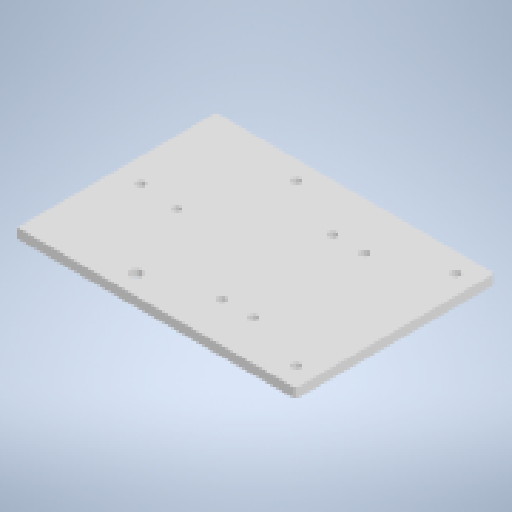
# Autodesk Inventor part: C beam gantry (big side y axis)
Saved by Autodesk Inventor 2023.2 (Build 272271000, 271)
## iProperties
Created: 2023-03-20
Part Number: C beam gantry (big side y axis)
Material: Generic
Document SubType Name: Modeling
Designer: dmargari
Density: 1 g/cm^3
Appearance: Default
Author: dmargari
Autodesk Inventor part; units mm, degrees
ref_plane "YZ Plane" through (0, 0, 0) normal (1, 0, 0) x (0, 1, 0)
ref_plane "XZ Plane" through (0, 0, 0) normal (0, 1, 0) x (-1, 0, 0)
ref_plane "XY Plane" through (0, 0, 0) normal (0, 0, 1) x (1, 0, 0)
sketch "Sketch1" plane through (0, 0, 0) normal (0, 1, 0) x (-1, 0, 0)
  line L0 (185.292, -262.2018) -> (60.092, -262.2018)
  line L1 (60.092, -262.2018) -> (60.092, -387.4018)
  line L2 (60.092, -387.4018) -> (185.292, -387.4018)
  line L3 (185.292, -387.4018) -> (185.292, -262.2018) construction
  line L4 (172.992, -262.2018) -> (172.992, -387.4018) construction
  line L5 (72.392, -262.2018) -> (72.392, -387.4018) construction
  line L6 (185.292, -262.2018) -> (235.292, -262.2018)
  line L7 (235.292, -262.2018) -> (235.292, -387.4018)
  line L8 (235.292, -387.4018) -> (185.292, -387.4018)
  line L9 (197.26, -375.1018) -> (25.4497, -375.1018) construction
  line L10 (197.26, -274.5018) -> (25.4497, -274.5018) construction
  point P0 (0, 0)
  point P1 (-73.8984, 140.5937)
  point P2 (172.992, -375.1018)
  point P3 (72.392, -375.1018)
  point P4 (172.992, -274.5018)
  point P5 (72.392, -274.5018)
  dimension "d0" = 125.2
  dimension "d1" = 125.2
  dimension "d2" = 12.3
  dimension "d3" = 12.3
  dimension "d8" = 50
  dimension "d35" = 12.3
  dimension "d36" = 100.6
  constraints: 22 end point, 13 point on line, 4 horizontal, 4 perpendicular, 2 parallel, 1 collinear
  measures "d0" distance of L2.end L1.end
  measures "d1" distance of L1.end L0.end
  measures "d2" distance between parallel lines of L1 L5
  measures "d3" distance between parallel lines of L3 L4
  measures "d8" distance of L0.start L6.end
  measures "d35" distance between parallel lines of L2 L9
  measures "d36" distance between parallel lines of L9 L10
extrude "Extrusion1" add sketch "Sketch1" along normal blind 6
fillet "Fillet1" radius 2 2 edges at (-60.092, 3, -262.2018) (-60.092, 3, -387.4018)
sketch "Sketch2" plane through (0, 6, 0) normal (0, 1, 0) x (1, 0, 0)
  line L0 (-235.292, 387.4018) -> (-235.292, 262.2018) construction
  line L1 (-235.292, 324.8018) -> (-60.092, 324.8018) construction
  line L2 (-60.092, 264.2018) -> (-60.092, 385.4018) construction
  line L3 (-235.192, 314.8018) -> (-30.192, 314.8018) construction
  line L4 (-235.192, 334.8018) -> (-30.192, 334.8018) construction
  line L5 (-235.292, 262.2018) -> (-62.092, 262.2018) construction
  line L6 (-220.292, 262.2018) -> (-220.292, 387.4018) construction
  line L7 (-62.092, 387.4018) -> (-235.292, 387.4018) construction
  line L8 (-195.292, 257.4018) -> (-195.292, 387.4018) construction
  point P0 (0, 0)
  point P1 (-220.292, 324.8018)
  point P2 (-195.292, 322.4018)
  dimension "d12" = 10
  dimension "d13" = 10
  dimension "d14" = 15
  dimension "d15" = 25
  constraints: 10 end point, 4 midpoint, 2 parallel, 2 point on line, 2 vertical
  measures "d12" distance between parallel lines of L1 L3
  measures "d13" distance between parallel lines of L1 L4
  measures "d14" distance between parallel lines of L0 L6
  measures "d15" distance between parallel lines of L8 L6
hole "Hole1" at (-220.292, 6, -324.8018) at (-195.292, 6, -322.4018) direction (0, -1, 0) diameter 5.1 end through all
sketch "Sketch3" plane through (0, 6, 0) normal (0, 1, 0) x (1, 0, 0)
  circle A0 centre (-112.092, 292.2018) radius 2.55 projected
  circle A1 centre (-132.092, 292.2018) radius 2.55 projected
  circle A2 centre (-132.092, 357.4018) radius 2.55 projected
  circle A3 centre (-112.092, 357.4018) radius 2.55 projected
  point P0 (0, 0)
hole "Hole2" at (-132.092, 6, -292.2018) at (-112.092, 6, -292.2018) at (-112.092, 6, -357.4018) at (-132.092, 6, -357.4018) direction (0, -1, 0) diameter 5.1 end through all
hole "Hole3" at (-172.992, 0, -274.5018) direction (0, 1, 0) diameter 7.2 end through all
hole "Hole4" at (-172.992, 0, -375.1018) at (-72.392, 0, -375.1018) at (-72.392, 0, -274.5018) direction (0, 1, 0) diameter 5.1 end through all
body "Solid1"
